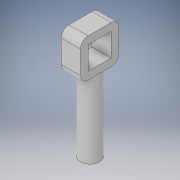
# Autodesk Inventor part: roka2
Saved by Autodesk Inventor 2019 (Build 230136000, 136)
## iProperties
Created: 2020-07-24
Part Number: roka2
Material: Generic
Document SubType Name: Modeling
Designer: lukad
Density: 1 g/cm^3
Appearance: Default
Author: lukad
Autodesk Inventor part; units mm, degrees
ref_plane "YZ Plane" through (0, 0, 0) normal (1, 0, 0) x (0, 1, 0)
ref_plane "XZ Plane" through (0, 0, 0) normal (0, 1, 0) x (-1, 0, 0)
ref_plane "XY Plane" through (0, 0, 0) normal (0, 0, 1) x (1, 0, 0)
sketch "Sketch1" plane through (0, 0, 0) normal (1, 0, 0) x (0, 1, 0)
  line L0 (6, 6) -> (0, 6)
  line L1 (0, 6) -> (0, 0)
  line L2 (0, 0) -> (6, 0)
  line L3 (6, 0) -> (6, 6)
  line L4 (-2, 8) -> (8, 8)
  line L5 (8, 8) -> (8, -2)
  line L6 (8, -2) -> (-2, -2)
  line L7 (-2, -2) -> (-2, 8)
  dimension "d0" = 6
  dimension "d1" = 6
  dimension "d2" = 2
  dimension "d3" = 10
  dimension "d4" = 10
  dimension "d5" = 2
  constraints: 16 end point, 4 parallel, 2 horizontal, 2 perpendicular
  measures "d0" distance between parallel lines of L1 L3
  measures "d1" distance between parallel lines of L2 L0
  measures "d2" distance between parallel lines of L5 L3
  measures "d3" distance between parallel lines of L7 L5
  measures "d4" distance between parallel lines of L6 L4
  measures "d5" distance between parallel lines of L6 L2
extrude "Extrusion1" add sketch "Sketch1" along normal blind 5
sketch "Sketch2" plane through (0, -2, -2) normal (0, -1, 0) x (1, 0, 0)
  circle A0 centre (2.5, 5) radius 2.5
  line L0 (0, 10) -> (5, 10) projected
  line L1 (5, 10) -> (5, 0) projected
  point P0 (0, 2)
  dimension "d8" = 5
  dimension "d9" = 5
  dimension "d10" = 2.5
  constraints: 1 centre point
  measures "d8" diameter of A0
  measures "d9" distance from line of L0 A0.centre
  measures "d10" distance from line of L1 A0.centre
extrude "Extrusion2" add sketch "Sketch2" along normal blind 20
fillet "Fillet1" radius 2 4 edges at (2.5, 8, 8) (2.5, 8, -2) (2.5, -2, 8) (2.5, -2, -2)
body "Solid1"
